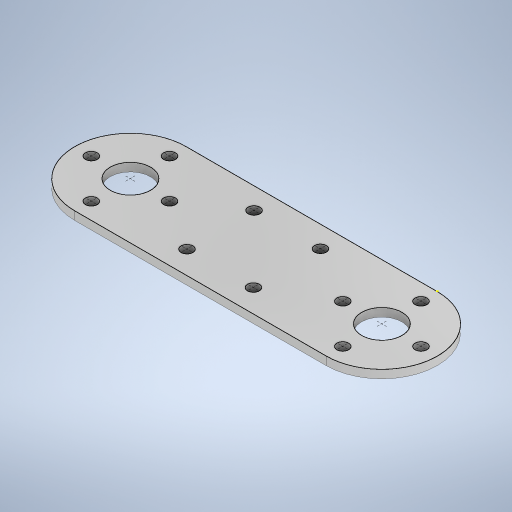
# Autodesk Inventor part: axis_3_bottom_frame(top)
Saved by Autodesk Inventor 2024.2 (Build 282272000, 272)
## iProperties
Created: 2023-12-25
Part Number: axis_3_bottom_frame(top)
Material: Aluminum 6061-AHC
Document SubType Name: Modeling
Designer: chanh
Density: 2.7 g/cm^3
Appearance: Aluminum - Dark
Author: chanh
Autodesk Inventor part; units mm, degrees
ref_plane "YZ Plane" through (0, 0, 0) normal (1, 0, 0) x (0, 1, 0)
ref_plane "XZ Plane" through (0, 0, 0) normal (0, 1, 0) x (-1, 0, 0)
ref_plane "XY Plane" through (0, 0, 0) normal (0, 0, 1) x (1, 0, 0)
sketch "Sketch1" plane through (0, 0, 0) normal (0, 1, 0) x (-1, 0, 0)
  circle A0 centre (29.0135, 3.825) radius 1.05
  circle A1 centre (17.1265, 3.825) radius 1.05
  circle A2 centre (17.1265, 15.825) radius 1.05
  circle A3 centre (29.0135, 15.825) radius 1.05
  circle A4 centre (0, 9.96) radius 3.6
  circle A5 centre (45, 9.96) radius 3.6
  circle A6 centre (0, 16.96) radius 1.05
  circle A7 centre (-7, 9.96) radius 1.05
  circle A8 centre (0, 2.96) radius 1.05
  circle A9 centre (7, 9.96) radius 1.05
  circle A10 centre (45, 16.96) radius 1.05
  circle A11 centre (38, 9.96) radius 1.05
  circle A12 centre (45, 2.96) radius 1.05
  circle A13 centre (52, 9.96) radius 1.05
  arc A14 (45, 0) -> (45, 19.92) centre (45, 9.96) ccw
  line L0 (0, 19.92) -> (45, 19.92)
  arc A15 (0, 19.92) -> (0, 0) centre (0, 9.96) ccw
  line L1 (45, 0) -> (0, 0)
  point P0 (0, 0)
  constraints: 16 centre point, 4 end point, 4 point on circle, 2 horizontal, 35 other
extrude "Extrusion1" add sketch "Sketch1" against normal blind 1.5
body "Solid1"
